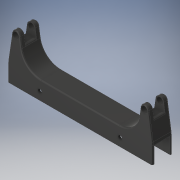
# Autodesk Inventor part: 2point_fixture
Saved by Autodesk Inventor 2019.4 (Build 234330000, 330)
## iProperties
Created: 2020-10-04
Part Number: 2point_fixture
Material: Generic
Document SubType Name: Modeling
Designer: deanv
Density: 1 g/cm^3
Appearance: Smooth - Black
Author: deanv
Autodesk Inventor part; units mm, degrees
ref_plane "YZ Plane" through (0, 0, 0) normal (1, 0, 0) x (0, 1, 0)
ref_plane "XZ Plane" through (0, 0, 0) normal (0, 1, 0) x (-1, 0, 0)
ref_plane "XY Plane" through (0, 0, 0) normal (0, 0, 1) x (1, 0, 0)
sketch "Sketch1" plane through (0, 0, 0) normal (0, 0, 1) x (1, 0, 0)
  line L0 (-90, -27.5) -> (90, -27.5) construction
  line L1 (90, -27.5) -> (90, 27.5) construction
  line L2 (90, 27.5) -> (-90, 27.5) construction
  line L3 (-90, 27.5) -> (-90, -27.5) construction
  line L4 (-90, -27.5) -> (90, 27.5) construction
  line L5 (90, -27.5) -> (-90, 27.5) construction
  line L6 (-90, -27.5) -> (90, -27.5)
  line L7 (90, -27.5) -> (90, -7.5)
  line L8 (90, -7.5) -> (-90, -7.5)
  line L9 (-90, -7.5) -> (-90, -27.5)
  line L10 (-80, -27.5) -> (80, -27.5) construction
  line L11 (80, -27.5) -> (80, 27.5) construction
  line L12 (80, 27.5) -> (-80, 27.5) construction
  line L13 (-80, 27.5) -> (-80, -27.5) construction
  circle A0 centre (-80, 27.5) radius 5 construction
  circle A1 centre (80, 27.5) radius 5 construction
  line L14 (-90, -7.5) -> (90, -7.5)
  line L15 (90, -7.5) -> (90, -5)
  line L16 (90, -5) -> (-90, -5)
  line L17 (-90, -5) -> (-90, -7.5)
  line L18 (-90, -5) -> (-84.943165, 28.251743) construction
  line L19 (-70, -5) -> (-75.056835, 28.251743) construction
  line L20 (90, -5) -> (84.943165, 28.251743) construction
  line L21 (70, -5) -> (75.056835, 28.251743) construction
  line L22 (-90, -5) -> (90, -5)
  line L23 (90, -5) -> (84.943165, 28.251743)
  arc A2 (84.943165, 28.251743) -> (75.056835, 28.251743) centre (80, 27.5) ccw
  line L24 (75.056835, 28.251743) -> (70, -5)
  line L25 (70, -5) -> (-70, -5)
  line L26 (-70, -5) -> (-75.056835, 28.251743)
  arc A3 (-75.056835, 28.251743) -> (-84.943165, 28.251743) centre (-80, 27.5) ccw
  line L27 (-84.943165, 28.251743) -> (-90, -5)
  circle A4 centre (-80, 27.5) radius 11
  circle A5 centre (80, 27.5) radius 11
  line L28 (-90, -7.5) -> (90, -27.5) construction
  line L29 (-90, -27.5) -> (90, -7.5) construction
  line L30 (-90, -17.5) -> (90, -17.5) construction
  line L31 (0, -27.5) -> (0, 0) construction
  line L32 (-80, -5) -> (80, -5)
  line L33 (80, -5) -> (80, 15)
  line L34 (80, 15) -> (-80, 15)
  line L35 (-80, 15) -> (-80, -5)
  point P0 (-50, -17.5)
  point P1 (50, -17.5)
  dimension "d0" = 180
  dimension "d1" = 55
  dimension "d2" = 180
  dimension "d3" = 20
  dimension "d4" = 160
  dimension "d5" = 10
  dimension "d6" = 10
  dimension "d7" = 10
  dimension "d10" = 180
  dimension "d11" = 2.5
  dimension "d12" = 10
  dimension "d13" = 10
  dimension "d18" = 22
  dimension "d19" = 22
  dimension "d34" = 50
  dimension "d35" = 100
  dimension "d45" = 20
  constraints: 72 end point, 10 parallel, 9 point on line, 9 tangent, 8 point on circle, 6 centre point, 6 coincident, 5 collinear, 5 horizontal, 5 midpoint, 5 perpendicular, 1 concentric
  measures "d0" distance of L2.end L1.end
  measures "d1" distance of L1.end L0.end
  measures "d2" distance of L8.end L7.end
  measures "d3" distance of L7.end L6.end
  measures "d4" distance between parallel lines of L11 L13
  measures "d5" distance between parallel lines of L3 L13
  measures "d6" diameter of A0
  measures "d7" diameter of A1
  measures "d10" distance of L16.end L15.end
  measures "d11" distance between parallel lines of L8 L16
  measures "d12" distance from line of L11 L21.start
  measures "d13" distance from line of L13 L19.start
  measures "d18" diameter of A4
  measures "d19" diameter of A5
  measures "d34" distance from line of L31 point (-50, -17.5)
  measures "d35" distance of point (50, -17.5) point (-50, -17.5)
  measures "d45" distance between parallel lines of L32 L34
extrude "Extrusion1" add sketch "Sketch1" along normal mid plane 25 contours L17 L16 L15 L8 | L27 A4 L26 L34 L35 L16 | L16 L33 L34 L24 A5 L23 | L35 L34 L26 L16 | L27 A3 L26 A4 | L16 L24 L34 L33 | A5 L24 A2 L23 picked at (-79.544473, 24.362902) picked at (80.455527, 24.362902)
extrude "Extrusion2" add sketch "Sketch1" along normal mid plane 25 contours L9 L8 L7 L6
extrude "Extrusion3" cut sketch "Sketch1" along normal mid plane 14 contours A4 L26 A3 L27 | L27 A3 L26 A4 | A5 L24 A2 L23 | L23 A2 L24 A5
hole "Hole1" at (-80, 27.5, 0) at (80, 27.5, 0) direction (0, 0, -1) diameter 8 end through all both
sketch "Sketch2" plane through (90, -5, 12.5) normal (1, 0, 0) x (0, 0, -1)
  line L0 (25, 0) -> (0, 0) projected
  line L1 (0, -22.5) -> (0, 0) projected
  line L2 (0, 0) -> (0, -22.5) construction
  line L3 (0, 0) -> (25, 0) construction
  line L4 (25, 0) -> (25, -22.5) construction
  line L5 (25, -22.5) -> (0, -22.5) construction
  line L6 (0, -22.5) -> (0, 0) construction
  line L7 (2.5, -22.5) -> (22.5, -22.5)
  line L8 (22.5, -22.5) -> (22.5, -2.5)
  line L9 (22.5, -2.5) -> (2.5, -2.5)
  line L10 (2.5, -2.5) -> (2.5, -22.5)
  point P0 (12.5, 5)
  dimension "d29" = 20
  dimension "d30" = 2.5
  dimension "d31" = 2.5
  constraints: 16 end point, 4 parallel, 2 horizontal, 2 perpendicular, 1 point on line
  measures "d29" distance between parallel lines of L8 L10
  measures "d30" distance between parallel lines of L1 L10
  measures "d31" distance between parallel lines of L0 L9
extrude "Extrusion4" cut sketch "Sketch2" against normal blind 180
hole "Hole2" at (-50, -17.5, 0) at (50, -17.5, 0) direction (0, 0, -1) diameter 5 end through all both
fillet "Fillet2" radius 25 2 edges at (90, -5, 0) (-90, -5, 0)
fillet "Fillet3" radius 25 2 edges at (-70, -5, 0) (70, -5, 0)
fillet "Fillet4" radius 1.5 26 edges at (-89.9289, -5.0054, 12.5) (-90, -17.1951, 12.5) (-80, 32.5, 12.5) (-74.1436, 22.2465, 12.5) (-64.8092, 1.0399, 12.5) (0, -5, 12.5) (64.8092, 1.0399, 12.5) (74.1436, 22.2465, 12.5) (80, 32.5, 12.5) (87.3295, 12.5602, 12.5) (89.9289, -5.0054, 12.5) (90, -17.1951, 12.5) (-87.3295, 12.5602, 12.5) (-64.8092, 1.0399, -12.5) (0, -5, -12.5) (64.8092, 1.0399, -12.5) (74.1436, 22.2465, -12.5) (80, 32.5, -12.5) (87.3295, 12.5602, -12.5) (89.9289, -5.0054, -12.5) (90, -17.1951, -12.5) (-80, 32.5, -12.5) (-87.3295, 12.5602, -12.5) (-89.9289, -5.0054, -12.5) (-90, -17.1951, -12.5) (-74.1436, 22.2465, -12.5)
fillet "Fillet5" radius 1.5 4 edges at (86.4163, 18.5652, 0) (73.5837, 18.5652, 0) (-73.5837, 18.5652, 0) (-86.4163, 18.5652, 0)
equation "\"d5\" = -0.5 * d4 + 0.5 * d0"
equation "\"d10\" = d0"
equation "\"d12\" = d5"
equation "\"d13\" = d5"
equation "\"d31\" = d30"
body "Solid1"
